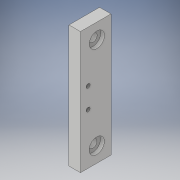
# Autodesk Inventor part: NeedleValvePanel V1
Saved by Autodesk Inventor 2019 (Build 230136000, 136)
## iProperties
Created: 2019-01-04
Part Number: NeedleValvePanel V1
Material: Generic
Document SubType Name: Modeling
Designer: dewanlab
Density: 1 g/cm^3
Appearance: Default
Author: dewanlab
Autodesk Inventor part; units mm, degrees
ref_plane "YZ Plane" through (0, 0, 0) normal (1, 0, 0) x (0, 1, 0)
ref_plane "XZ Plane" through (0, 0, 0) normal (0, 1, 0) x (-1, 0, 0)
ref_plane "XY Plane" through (0, 0, 0) normal (0, 0, 1) x (1, 0, 0)
sketch "Sketch1" plane through (0, 0, 0) normal (1, 0, 0) x (0, 1, 0)
  line L0 (0, 0) -> (101.6, 0)
  line L1 (101.6, 0) -> (101.6, -25.4)
  line L2 (101.6, -25.4) -> (0, -25.4)
  line L3 (0, -25.4) -> (0, 0)
  point P0 (95.25, -12.7)
  point P1 (6.35, -12.7)
  dimension "d0" = 25.4
  dimension "d1" = 101.6
  dimension "d4" = 6.35
  dimension "d5" = 12.7
  dimension "d6" = 6.35
  constraints: 8 end point, 2 parallel, 1 horizontal, 1 perpendicular
  measures "d0" distance between parallel lines of L2 L0
  measures "d1" distance from line of L3 L1.end
  measures "d4" distance from line of point (95.25, -12.7) L1
  measures "d5" distance from line of L0 point (95.25, -12.7)
  measures "d6" distance from line of L3 point (6.35, -12.7)
extrude "Extrusion1" add sketch "Sketch1" along normal blind 9.525
sketch "Sketch2" plane through (9.525, 0, 0) normal (1, 0, 0) x (0, 0, -1)
  line L0 (25.4, 101.6) -> (0, 101.6) projected
  point P0 (0, 0)
  point P1 (13.6787, 88.9)
  dimension "d22" = 12.7
  measures "d22" distance from line of L0 point (13.679, 88.9)
hole "Hole1" at (9.525, 88.9, -13.6787) direction (-1, 0, 0) diameter 6.7564 end through all counterbore diameter 12.7 counterbore depth 3.175
sketch "Sketch3" plane through (9.525, 0, 0) normal (1, 0, 0) x (0, 0, -1)
  line L0 (0, 0) -> (25.4, 0) projected
  point P0 (13.5273, 12.7)
  dimension "d21" = 12.7
  measures "d21" distance from line of L0 point (13.527, 12.7)
hole "Hole2" at (9.525, 12.7, -13.5273) direction (-1, 0, 0) diameter 6.7564 end through all counterbore diameter 12.7 counterbore depth 3.175
sketch "Sketch4" plane through (9.525, 0, 0) normal (1, 0, 0) x (0, 0, -1)
  line L0 (0, 101.6) -> (0, 0) projected
  line L1 (25.4, 101.6) -> (0, 101.6) projected
  point P0 (6.35, 59.3)
  dimension "d30" = 6.35
  dimension "d31" = 42.3
  measures "d30" distance from line of L0 point (6.35, 59.3)
  measures "d31" distance from line of L1 point (6.35, 59.3)
hole "Hole3" at (9.525, 59.3, -6.35) direction (-1, 0, 0) diameter 3.302 end through all thread size "8-32 UNC" class "2B" standard "ANSI Unified Screw Threads"
sketch "Sketch5" plane through (9.525, 0, 0) normal (1, 0, 0) x (0, 0, -1)
  line L0 (0, 0) -> (25.4, 0) projected
  line L1 (0, 101.6) -> (0, 0) projected
  point P0 (6.35, 42.3)
  dimension "d39" = 42.3
  dimension "d40" = 6.35
  measures "d39" distance from line of L0 point (6.35, 42.3)
  measures "d40" distance from line of L1 point (6.35, 42.3)
hole "Hole4" at (9.525, 42.3, -6.35) direction (-1, 0, 0) diameter 3.302 end through all thread size "8-32 UNC" class "2B" standard "ANSI Unified Screw Threads"
body "Solid1"
